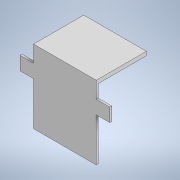
# Autodesk Inventor part: shell 6.0 cover
Saved by Autodesk Inventor 2020.2 (Build 242310000, 310)
## iProperties
Created: 2020-03-16
Part Number: shell 6.0 cover
Material: Generic
Document SubType Name: Modeling
Designer: ColinP
Density: 1 g/cm^3
Appearance: Default
Author: ColinP
Autodesk Inventor part; units mm, degrees
ref_plane "YZ Plane" through (0, 0, 0) normal (1, 0, 0) x (0, 1, 0)
ref_plane "XZ Plane" through (0, 0, 0) normal (0, 1, 0) x (-1, 0, 0)
ref_plane "XY Plane" through (0, 0, 0) normal (0, 0, 1) x (1, 0, 0)
sketch "Sketch1" plane through (0, 0, 0) normal (0, 0, 1) x (1, 0, 0)
  line L0 (-10.2966, 10.8783) -> (22.1834, 10.8783)
  line L1 (22.1834, 10.8783) -> (22.1834, -25.1217)
  line L2 (22.1834, -25.1217) -> (-10.2966, -25.1217)
  line L3 (-10.2966, -25.1217) -> (-10.2966, 10.8783)
  line L4 (-10.2966, -25.1217) -> (-10.2966, -2.6417)
  line L5 (-10.2966, -2.6417) -> (-17.2966, -2.6417)
  line L6 (-17.2966, -2.6417) -> (-17.2966, 4.3583)
  line L7 (-17.2966, 4.3583) -> (-10.2966, 4.3583)
  line L8 (22.1834, 4.3583) -> (29.1834, 4.3583)
  line L9 (29.1834, 4.3583) -> (29.1834, -2.6417)
  line L10 (29.1834, -2.6417) -> (22.1834, -2.6417)
  line L11 (-10.2966, 10.8783) -> (-10.2966, 12.8783)
  line L12 (-10.2966, 12.8783) -> (22.1834, 12.8783)
  line L13 (22.1834, 12.8783) -> (22.1834, 10.8783)
  point P0 (0, 0)
  dimension "d0" = 32.48
  dimension "d1" = 36
  dimension "d2" = 22.48
  dimension "d3" = 7
  dimension "d4" = 90
  dimension "d5" = 7
  dimension "d6" = 7
  dimension "d7" = 2
  constraints: 28 end point, 9 point on line, 7 perpendicular, 2 parallel, 1 horizontal
  measures "d0" distance of L1.end L2.end
  measures "d1" distance of L0.end L1.end
  measures "d2" distance of L2.end L4.end
  measures "d3" distance of L4.end L5.end
  measures "d4" angle of L5 L4
  measures "d5" distance of L5.end L6.end
  measures "d6" distance of L8.start L8.end
  measures "d7" distance of L0.start L11.end
extrude "Extrusion1" add sketch "Sketch1" along normal blind 1
extrude "Extrusion2" add sketch "Sketch1" against normal blind 25 contours L11 L12 L13 L0
body "Solid1"
